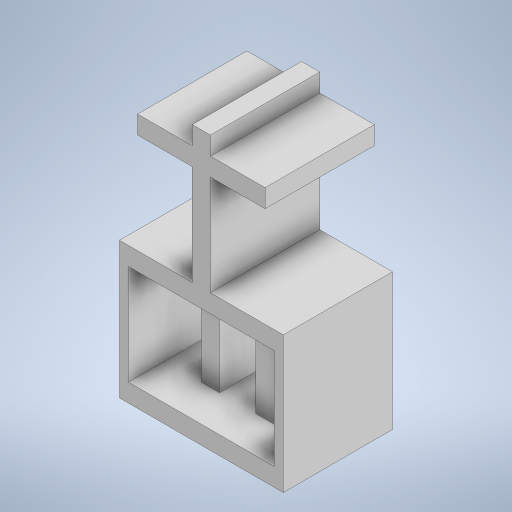
# Autodesk Inventor part: 팔
Saved by Autodesk Inventor 2024 (Build 280153000, 153)
## iProperties
Created: 2023-05-04
Part Number: 팔
Material: 일반
Document SubType Name: Modeling
Designer: hjcho
Density: 1 g/cm^3
Appearance: 기본값
Author: hjcho
Autodesk Inventor part; units mm, degrees
ref_plane "YZ Plane" through (0, 0, 0) normal (1, 0, 0) x (0, 1, 0)
ref_plane "XZ Plane" through (0, 0, 0) normal (0, 1, 0) x (-1, 0, 0)
ref_plane "XY Plane" through (0, 0, 0) normal (0, 0, 1) x (1, 0, 0)
sketch "스케치1" plane through (0, 0, 0) normal (0, 0, 1) x (1, 0, 0)
  line L0 (0, 0) -> (0, 150)
  line L1 (45, 0) -> (-45, 0)
  line L2 (-45, 0) -> (-45, 10)
  line L3 (-45, 10) -> (45, 10)
  line L4 (45, 10) -> (45, 0)
  line L5 (45, 0) -> (-45, 10) construction
  line L6 (-45, 0) -> (45, 10) construction
  line L7 (-35, 130) -> (35, 130)
  line L8 (35, 130) -> (35, 140)
  line L9 (35, 140) -> (-35, 140)
  line L10 (-35, 140) -> (-35, 130)
  line L11 (-35, 130) -> (35, 140) construction
  line L12 (35, 130) -> (-35, 140) construction
  line L13 (-40, 65) -> (40, 65)
  line L14 (40, 65) -> (40, 75)
  line L15 (40, 75) -> (-40, 75)
  line L16 (-40, 75) -> (-40, 65)
  line L17 (-40, 65) -> (40, 75) construction
  line L18 (40, 65) -> (-40, 75) construction
  line L19 (5, 150) -> (-5, 150)
  line L20 (-5, 0) -> (5, 0)
  line L21 (-45, 10) -> (-40, 10)
  line L22 (-40, 10) -> (-40, 75)
  line L23 (-40, 75) -> (-45, 75)
  line L24 (-45, 75) -> (-45, 10)
  line L25 (45, 10) -> (40, 10)
  line L26 (40, 10) -> (40, 75)
  line L27 (40, 75) -> (45, 75)
  line L28 (45, 75) -> (45, 10)
  line L29 (5, 0) -> (5, 10)
  line L30 (5, 65) -> (5, 150)
  line L31 (-5, 150) -> (-5, 65)
  line L32 (-5, 10) -> (-5, 0)
  line L33 (0, 10) -> (10, 10)
  line L34 (10, 10) -> (10, 65)
  line L35 (10, 65) -> (0, 65)
  line L36 (0, 65) -> (0, 10)
  line L37 (0, 10) -> (-10, 10)
  line L38 (-10, 10) -> (-10, 65)
  line L39 (-10, 65) -> (0, 65)
  line L40 (0, 65) -> (0, 10)
  line L41 (-10, 65) -> (-20, 65)
  line L42 (-20, 65) -> (-20, 10)
  line L43 (-20, 10) -> (-10, 10)
  line L44 (-10, 10) -> (-10, 65)
  line L45 (10, 65) -> (20, 65)
  line L46 (20, 65) -> (20, 10)
  line L47 (20, 10) -> (10, 10)
  line L48 (10, 10) -> (10, 65)
  point P0 (0, 5)
  point P1 (0, 135)
  point P2 (0, 70)
  point P3 (-5, 140)
  point P4 (5, 140)
  point P5 (-5, 75)
  point P6 (5, 75)
  point P7 (-5, 130)
  point P8 (5, 130)
  dimension "d16" = 150
  dimension "d17" = 90
  dimension "d18" = 10
  dimension "d22" = 70
  dimension "d23" = 10
  dimension "d25" = 80
  dimension "d26" = 10
  dimension "d27" = 55
  dimension "d28" = 55
  dimension "d29" = 10
  dimension "d30" = 150
  dimension "d35" = 10
  dimension "d36" = 10
  dimension "d37" = 10
  dimension "d38" = 10
  constraints: 98 end point, 23 parallel, 11 perpendicular, 10 horizontal, 8 point on line, 7 midpoint, 2 vertical
  measures "d16" distance of L0.start L0.end
  measures "d17" distance of L2.end L3.end
  measures "d18" distance of L1.end L2.end
  measures "d22" distance of L9.end L8.end
  measures "d23" distance of L8.end L7.end
  measures "d25" distance of L15.end L14.end
  measures "d26" distance of L14.end L13.end
  measures "d27" distance between parallel lines of L3 L13
  measures "d28" distance between parallel lines of L15 L7
  measures "d29" distance of L20.end L20.start
  measures "d30" distance of L20.start L19.end
  measures "d35" distance of L35.end L34.end
  measures "d36" distance of L38.end L39.end
  measures "d37" distance of L43.end L42.end
  measures "d38" distance of L46.end L47.end
extrude "돌출1" add sketch "스케치1" along normal blind 30 and the other way blind 30 contours L1 L32 L3 L0 | L0 L3 L29 L1 | L29 L3 L4 L1 | L1 L2 L3 L32 | L13 L31 L15 L0 | L0 L15 L30 L13 | L15 L31 L7 L0 | L0 L7 L30 L15 | L13 L16 L15 L31 | L30 L15 L14 L13 | L7 L31 L9 L0 | L0 L9 L30 L7 | L9 L31 L19 L0 | L0 L19 L30 L9 | L7 L10 L9 L31 | L30 L9 L8 L7
extrude "돌출2" add sketch "스케치1" along normal blind 30 and the other way blind 30 contours L3 L26 L14 L27 L28 | L24 L23 L16 L22 L3
extrude "돌출3" add sketch "스케치1" along normal blind 10 and the other way blind 10 contours L3 L42 L13 L38 | L34 L13 L46 L3
